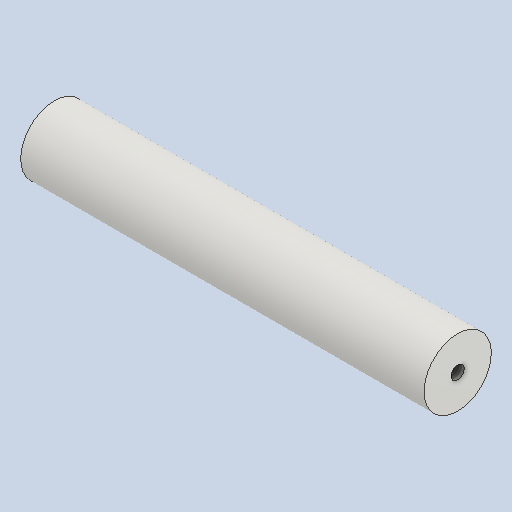
# Autodesk Inventor part: Wał
Saved by Autodesk Inventor 2023 (Build 270158000, 158)
## iProperties
CustomPartVersion: 1
Created: 2023-04-10
Part Number: Wał
Material: Steel
Document SubType Name: Modeling
Designer: Wiktor
Density: 7.85 g/cm^3
Appearance: Steel
Mass: 578.004 g
Surface Area: 127.627 cm^2
Volume: 73.6311 cm^3
Length: 150,000 mm
Author: Wiktor
Autodesk Inventor part; units mm, degrees
ref_plane "Płaszczyzna początkowa" through (0, 0, 0) normal (1, 0, 0) x (0, 1, 0)
ref_plane "XZ Plane" through (0, 0, 0) normal (0, 1, 0) x (-1, 0, 0)
ref_plane "XY Plane" through (0, 0, 0) normal (0, 0, 1) x (1, 0, 0)
sketch "Szkic główny" plane through (0, 0, 0) normal (0, 0, 1) x (1, 0, 0)
  line L0 (0, 0) -> (150, 0)
  line L1 (0, 0) -> (0, 12.5)
  line L2 (150, 12.5) -> (150, 0)
  line L3 (0, 12.5) -> (150, 12.5)
  dimension "d3" = 25
  constraints: 8 end point, 3 horizontal, 2 vertical
  measures "d3" diameter of L3 L0
revolve "Obrót1" add sketch "Szkic główny" angle 360 about axis through (0, 0, 0) along (1, 0, 0)
sketch "Szkic3" plane through (0, 0, 0) normal (-1, 0, 0) x (0, 0, 1)
  point P0 (0, 0)
hole "Otwór1" at (0, 0, 0) direction (1, 0, 0) diameter 4.917 depth 19 tip angle 120 thread size "M6x1" class "6H" standard "ISO Metric profile"
sketch "Szkic4" plane through (150, 0, 0) normal (1, 0, 0) x (0, 0, -1)
  point P0 (0, 0)
hole "Otwór2" at (150, 0, 0) direction (-1, 0, 0) diameter 4.917 depth 18 tip angle 120 thread size "M6x1" class "6H" standard "ISO Metric profile"
equation "\"Length\" = 150"
